Autodesk Inventor part; units mm, degrees
(part 2 of 2)
sketch "Sketch28" plane through (0, 0, 0) normal (0, 0, 1) x (1, 0, 0)
  line L0 (36.6613, -0.85) -> (16.5, -0.85) construction
  line L1 (16.5, -3.9301) -> (16.5, -0.85) construction
  arc A0 (30.5468, -4.3971) -> (16.5, -3.9301) centre (23.1, -16.9) ccw construction
  line L2 (30.5468, -4.3971) -> (34.1307, -4.3971) construction
  line L3 (34.1307, -4.3971) -> (38, -8.2664) construction
  line L4 (38, -2.1887) -> (38, -8.2664) construction
  line L5 (38, -2.1887) -> (36.6613, -0.85) construction
  line L6 (42, -6.1887) -> (38, -2.1887) construction
  line L7 (38, -2.1887) -> (38, -8.2664) construction
  line L8 (38, -8.2664) -> (42, -12.2664) construction
  line L9 (42, -12.2664) -> (42, -6.1887) construction
  line L10 (34.1307, -29.4029) -> (36.4148, -32.95) construction
  line L11 (16.5, -32.95) -> (36.6613, -32.95) construction
  line L12 (38, -31.6113) -> (36.6613, -32.95) construction
  line L13 (38, -25.5336) -> (38, -31.6113) construction
  line L14 (34.1307, -29.4029) -> (38, -25.5336) construction
  line L15 (30.5468, -29.4029) -> (34.1307, -29.4029) construction
  arc A1 (16.5, -29.8699) -> (30.5468, -29.4029) centre (23.1, -16.9) ccw construction
  line L16 (16.5, -32.95) -> (16.5, -29.8699) construction
  line L17 (42, -21.5336) -> (38, -25.5336) construction
  line L18 (38, -25.5336) -> (38, -31.6113) construction
  line L19 (38, -31.6113) -> (42, -27.6113) construction
  line L20 (42, -27.6113) -> (42, -21.5336) construction
  line L21 (36.6613, -32.95) -> (42, -27.6113)
  line L22 (16.5, -32.95) -> (36.6613, -32.95) projected
  line L23 (36.4492, -32.95) -> (42, -27.3992)
  line L24 (36.4492, -32.95) -> (36.6613, -32.95)
  line L25 (46, -23.6113) -> (42, -27.6113) projected
  line L26 (42, -27.3992) -> (42, -27.6113)
  line L27 (-21.96, -16.9) -> (117.76, -16.9) construction
  line L28 (36.6613, -0.85) -> (42, -6.1887)
  line L29 (36.4492, -0.85) -> (42, -6.4008)
  line L30 (36.4492, -0.85) -> (36.6613, -0.85)
  line L31 (42, -6.4008) -> (42, -6.1887)
  point P0 (0, 0)
  point P1 (36.4148, -0.85)
  dimension "d65" = 0
  dimension "d66" = 3
  dimension "d144" = 0.15
  constraints: 16 end point, 3 symmetric about line, 2 point on line, 1 collinear, 1 horizontal, 1 parallel, 1 vertical
  measures "d144" distance between parallel lines of L19 L23
extrude "Extrusion28" cut sketch "Sketch28" against normal up to surface (11 mm away)
ref_plane "Work Plane5" through (6, -38.3, -33.8) normal (0, 0, -1) x (1, 0, 0)
ref_plane "Work Plane6" through (10.2, -29.4, -20.3) normal (0, 0, 1) x (-1, 0, 0)
ref_plane "Work Plane7" through (0, -33.8, -18) normal (0, 0, 1) x (-1, 0, 0)
body "Solid1"
